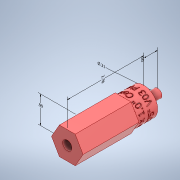
# Autodesk Inventor part: 1x8mmx1_1-inchHexShaft
Saved by Autodesk Inventor 2022.2 (Build 262287010, 287A)
## iProperties
Created: 2020-11-16
Part Number: 1x8mmx1_1-inchHexShaft
Material: PC/ABS Plastic
Document SubType Name: Modeling
Designer: robst
Density: 0.357273 g/cm^3
Appearance: Smooth - Red
Author: robst
Autodesk Inventor part; units mm, degrees
ref_plane "XZ Plane" through (0, 0, 0) normal (0, 1, 0) x (-1, 0, 0)
ref_plane "XY Plane" through (0, 0, 0) normal (0, 0, 1) x (1, 0, 0)
sketch "Sketch1" plane through (0, 0, 0) normal (0, 0, 1) x (1, 0, 0)
  line L0 (14.6647, 0) -> (7.3323, -12.7)
  line L1 (7.3323, -12.7) -> (-7.3323, -12.7)
  line L2 (-7.3323, -12.7) -> (-14.6647, 0)
  line L3 (-14.6647, 0) -> (-7.3323, 12.7)
  line L4 (-7.3323, 12.7) -> (7.3323, 12.7)
  line L5 (7.3323, 12.7) -> (14.6647, 0)
  point P0 (0, 0)
  point P1 (0, 0)
  dimension "d0" = 25.4
  constraints: 12 end point, 1 coincident, 1 horizontal, 13 other
  measures "d0" distance between parallel lines of L1 L4
extrude "Hex Portion" add sketch "Sketch1" along normal mid plane 51.435
sketch "Sketch2" plane through (0, 0, -25.7175) normal (0, 0, -1) x (-1, 0, 0)
  circle A0 centre (0, 0) radius 12.7
  dimension "d3" = 25.4
  constraints: 1 centre point, 1 coincident
  measures "d3" diameter of A0
extrude "Extrusion2" add sketch "Sketch2" along normal blind 19.05
thicken "Reduce Size of Hex Shaft" operation add thickness 0.0953 both sides no extend neighbours yes toward (-0.8660254, -0.5, 0) faces at (10.9985, 6.35, 8.5725) (0, 12.7, 8.5725) (10.9985, -6.35, 8.5725) (0, -12.7, 8.5725) (-10.9985, -6.35, 8.5725) (-10.9985, 6.35, 8.5725)
sketch "Sketch3" plane through (0, 0, -44.7675) normal (0, 0, -1) x (-1, 0, 0)
  circle A0 centre (0, 0) radius 4
  dimension "d14" = 8
  constraints: 1 centre point, 1 coincident
  measures "d14" diameter of A0
extrude "Extrusion3" add sketch "Sketch3" along normal blind 12.7
ref_plane "Work Plane1" through (12.7, 0, -25.7175) normal (1, 0, 0) x (0, 1, 0)
sketch "Sketch4" plane through (12.7, 0, -25.7175) normal (1, 0, 0) x (0, 1, 0)
  line L0 (-12.7, 0) -> (12.7, 0) projected
  line L1 (-12.7, -19.05) -> (12.7, -19.05) projected
  line L2 (-12.7, 0) -> (-12.7, -19.05) construction
  line L3 (-12.7, -9.525) -> (12.7, -9.525) construction
  line L4 (12.7, 0) -> (12.7, -19.05) construction
  line L5 (-33.1661, -6.985) -> (-35.6444, -6.985)
  line L6 (-35.6444, -6.985) -> (-35.6444, -6.4663)
  line L7 (-35.6444, -6.4663) -> (-34.7223, -6.4663)
  line L8 (-34.7223, -6.4663) -> (-34.7223, -3.0618)
  line L9 (-34.7223, -3.0618) -> (-35.6444, -3.0618)
  line L10 (-35.6444, -3.0618) -> (-35.6444, -2.5966)
  spline S0 degree 2 poles (-35.6444, -2.5966) (-35.1216, -2.5966) (-34.6276, -2.3002) (-34.5946, -1.8885) knots 0 0 0 1 2 2 2
  line L11 (-34.5946, -1.8885) -> (-34.0677, -1.8885)
  line L12 (-34.0677, -1.8885) -> (-34.0677, -6.4663)
  line L13 (-34.0677, -6.4663) -> (-33.1661, -6.4663)
  line L14 (-33.1661, -6.4663) -> (-33.1661, -6.985)
  line L15 (-31.4701, -1.6786) -> (-31.6183, -3.6546)
  line L16 (-31.6183, -3.6546) -> (-32.067, -3.6546)
  line L17 (-32.067, -3.6546) -> (-32.2152, -1.6786)
  line L18 (-32.2152, -1.6786) -> (-31.4701, -1.6786)
  line L19 (-30.1857, -1.6786) -> (-30.3339, -3.6546)
  line L20 (-30.3339, -3.6546) -> (-30.7826, -3.6546)
  line L21 (-30.7826, -3.6546) -> (-30.9308, -1.6786)
  line L22 (-30.9308, -1.6786) -> (-30.1857, -1.6786)
  line L23 (-24.1918, -6.985) -> (-24.978, -6.985)
  line L24 (-24.978, -6.985) -> (-25.9043, -5.5524)
  line L25 (-25.9043, -5.5524) -> (-26.8553, -6.985)
  line L26 (-26.8553, -6.985) -> (-27.5839, -6.985)
  line L27 (-27.5839, -6.985) -> (-26.2624, -5.0954)
  line L28 (-26.2624, -5.0954) -> (-27.5716, -3.1729)
  line L29 (-27.5716, -3.1729) -> (-26.7853, -3.1729)
  line L30 (-26.7853, -3.1729) -> (-25.8631, -4.5932)
  line L31 (-25.8631, -4.5932) -> (-24.9204, -3.1729)
  line L32 (-24.9204, -3.1729) -> (-24.1918, -3.1729)
  line L33 (-24.1918, -3.1729) -> (-25.505, -5.0543)
  line L34 (-25.505, -5.0543) -> (-24.1918, -6.985)
  spline S1 degree 2 poles (-20.0709, -7.1003) (-20.4497, -7.1003) (-21.0713, -6.8738) (-21.2895, -6.6639) knots 0 0 0 1 2 2 2
  spline S2 degree 2 poles (-21.2895, -6.6639) (-21.5036, -6.4581) (-21.7259, -5.8982) (-21.7259, -5.5812) knots 0 0 0 1 2 2 2
  spline S3 degree 2 poles (-21.7259, -5.5812) (-21.7259, -5.1695) (-21.2854, -4.4779) (-20.8655, -4.2721) knots 0 0 0 1 2 2 2
  line L35 (-20.8655, -4.2721) -> (-20.8655, -4.2515)
  spline S4 degree 2 poles (-20.8655, -4.2515) (-21.2401, -4.0333) (-21.6024, -3.5146) (-21.6024, -3.1277) knots 0 0 0 1 2 2 2
  spline S5 degree 2 poles (-21.6024, -3.1277) (-21.6024, -2.5554) (-20.7378, -1.7897) (-20.0709, -1.7897) knots 0 0 0 1 2 2 2
  spline S6 degree 2 poles (-20.0709, -1.7897) (-19.3793, -1.7897) (-18.5436, -2.5143) (-18.5436, -3.0824) knots 0 0 0 1 2 2 2
  spline S7 degree 2 poles (-18.5436, -3.0824) (-18.5436, -3.4241) (-18.943, -4.091) (-19.3176, -4.2803) knots 0 0 0 1 2 2 2
  line L36 (-19.3176, -4.2803) -> (-19.3176, -4.3009)
  spline S8 degree 2 poles (-19.3176, -4.3009) (-18.873, -4.5068) (-18.416, -5.0996) (-18.416, -5.5689) knots 0 0 0 1 2 2 2
  spline S9 degree 2 poles (-18.416, -5.5689) (-18.416, -6.2193) (-19.3629, -7.1003) (-20.0709, -7.1003) knots 0 0 0 1 2 2 2
  spline S10 degree 2 poles (-19.1159, -5.6347) (-19.1159, -5.3219) (-19.3629, -4.9514) (-19.7128, -4.762) knots 0 0 0 1 2 2 2
  spline S11 degree 2 poles (-19.7128, -4.762) (-19.8281, -4.6961) (-20.215, -4.5438) (-20.4579, -4.445) knots 0 0 0 1 2 2 2
  spline S12 degree 2 poles (-20.4579, -4.445) (-20.7378, -4.6303) (-21.0384, -5.1819) (-21.0384, -5.5318) knots 0 0 0 1 2 2 2
  spline S13 degree 2 poles (-21.0384, -5.5318) (-21.0384, -5.9929) (-20.4826, -6.5939) (-20.0627, -6.5939) knots 0 0 0 1 2 2 2
  spline S14 degree 2 poles (-20.0627, -6.5939) (-19.6346, -6.5939) (-19.1159, -6.0793) (-19.1159, -5.6347) knots 0 0 0 1 2 2 2
  spline S15 degree 2 poles (-19.2106, -3.0906) (-19.2106, -2.7489) (-19.6675, -2.292) (-20.0751, -2.292) knots 0 0 0 1 2 2 2
  spline S16 degree 2 poles (-20.0751, -2.292) (-20.4456, -2.292) (-20.919, -2.6995) (-20.919, -3.0494) knots 0 0 0 1 2 2 2
  spline S17 degree 2 poles (-20.919, -3.0494) (-20.919, -3.3006) (-20.6761, -3.6505) (-20.4332, -3.7904) knots 0 0 0 1 2 2 2
  spline S18 degree 2 poles (-20.4332, -3.7904) (-20.3303, -3.8481) (-19.8939, -4.0498) (-19.7169, -4.1074) knots 0 0 0 1 2 2 2
  spline S19 degree 2 poles (-19.7169, -4.1074) (-19.4205, -3.881) (-19.2106, -3.3994) (-19.2106, -3.0906) knots 0 0 0 1 2 2 2
  line L37 (-13.3772, -6.985) -> (-13.3772, -4.7785)
  spline S20 degree 2 poles (-13.3772, -4.7785) (-13.3772, -4.515) (-13.4184, -4.0663) (-13.4842, -3.9428) knots 0 0 0 1 2 2 2
  spline S21 degree 2 poles (-13.4842, -3.9428) (-13.5501, -3.8069) (-13.8012, -3.6752) (-14.0194, -3.6752) knots 0 0 0 1 2 2 2
  spline S22 degree 2 poles (-14.0194, -3.6752) (-14.217, -3.6752) (-14.6698, -3.9181) (-14.9086, -4.1486) knots 0 0 0 1 2 2 2
  spline S23 degree 2 poles (-14.9086, -4.1486) (-14.9045, -4.2062) (-14.8963, -4.3668) (-14.8963, -4.4738) knots 0 0 0 1 2 2 2
  line L38 (-14.8963, -4.4738) -> (-14.8963, -6.985)
  line L39 (-14.8963, -6.985) -> (-15.5385, -6.985)
  line L40 (-15.5385, -6.985) -> (-15.5385, -4.7785)
  spline S24 degree 2 poles (-15.5385, -4.7785) (-15.5385, -4.515) (-15.5796, -4.0663) (-15.6455, -3.9428) knots 0 0 0 1 2 2 2
  spline S25 degree 2 poles (-15.6455, -3.9428) (-15.7114, -3.8069) (-15.9625, -3.6752) (-16.1807, -3.6752) knots 0 0 0 1 2 2 2
  spline S26 degree 2 poles (-16.1807, -3.6752) (-16.3865, -3.6752) (-16.8435, -3.9345) (-17.0575, -4.1362) knots 0 0 0 1 2 2 2
  line L41 (-17.0575, -4.1362) -> (-17.0575, -6.985)
  line L42 (-17.0575, -6.985) -> (-17.6997, -6.985)
  line L43 (-17.6997, -6.985) -> (-17.6997, -3.1729)
  line L44 (-17.6997, -3.1729) -> (-17.0575, -3.1729)
  line L45 (-17.0575, -3.1729) -> (-17.0575, -3.5928)
  spline S27 degree 2 poles (-17.0575, -3.5928) (-16.8064, -3.3417) (-16.3124, -3.0659) (-16.016, -3.0659) knots 0 0 0 1 2 2 2
  spline S28 degree 2 poles (-16.016, -3.0659) (-15.6784, -3.0659) (-15.1556, -3.3747) (-15.0198, -3.7246) knots 0 0 0 1 2 2 2
  spline S29 degree 2 poles (-15.0198, -3.7246) (-14.7275, -3.3994) (-14.1758, -3.0659) (-13.8547, -3.0659) knots 0 0 0 1 2 2 2
  spline S30 degree 2 poles (-13.8547, -3.0659) (-13.6077, -3.0659) (-13.2043, -3.2182) (-13.0561, -3.3911) knots 0 0 0 1 2 2 2
  spline S31 degree 2 poles (-13.0561, -3.3911) (-12.9038, -3.564) (-12.735, -4.0827) (-12.735, -4.4738) knots 0 0 0 1 2 2 2
  line L46 (-12.735, -4.4738) -> (-12.735, -6.985)
  line L47 (-12.735, -6.985) -> (-13.3772, -6.985)
  line L48 (-7.5109, -6.985) -> (-7.5109, -4.7785)
  spline S32 degree 2 poles (-7.5109, -4.7785) (-7.5109, -4.515) (-7.5521, -4.0663) (-7.6179, -3.9428) knots 0 0 0 1 2 2 2
  spline S33 degree 2 poles (-7.6179, -3.9428) (-7.6838, -3.8069) (-7.9349, -3.6752) (-8.1531, -3.6752) knots 0 0 0 1 2 2 2
  spline S34 degree 2 poles (-8.1531, -3.6752) (-8.3507, -3.6752) (-8.8036, -3.9181) (-9.0423, -4.1486) knots 0 0 0 1 2 2 2
  spline S35 degree 2 poles (-9.0423, -4.1486) (-9.0382, -4.2062) (-9.03, -4.3668) (-9.03, -4.4738) knots 0 0 0 1 2 2 2
  line L49 (-9.03, -4.4738) -> (-9.03, -6.985)
  line L50 (-9.03, -6.985) -> (-9.6722, -6.985)
  line L51 (-9.6722, -6.985) -> (-9.6722, -4.7785)
  spline S36 degree 2 poles (-9.6722, -4.7785) (-9.6722, -4.515) (-9.7133, -4.0663) (-9.7792, -3.9428) knots 0 0 0 1 2 2 2
  spline S37 degree 2 poles (-9.7792, -3.9428) (-9.8451, -3.8069) (-10.0962, -3.6752) (-10.3144, -3.6752) knots 0 0 0 1 2 2 2
  spline S38 degree 2 poles (-10.3144, -3.6752) (-10.5202, -3.6752) (-10.9772, -3.9345) (-11.1912, -4.1362) knots 0 0 0 1 2 2 2
  line L52 (-11.1912, -4.1362) -> (-11.1912, -6.985)
  line L53 (-11.1912, -6.985) -> (-11.8334, -6.985)
  line L54 (-11.8334, -6.985) -> (-11.8334, -3.1729)
  line L55 (-11.8334, -3.1729) -> (-11.1912, -3.1729)
  line L56 (-11.1912, -3.1729) -> (-11.1912, -3.5928)
  spline S39 degree 2 poles (-11.1912, -3.5928) (-10.9401, -3.3417) (-10.4461, -3.0659) (-10.1497, -3.0659) knots 0 0 0 1 2 2 2
  spline S40 degree 2 poles (-10.1497, -3.0659) (-9.8121, -3.0659) (-9.2893, -3.3747) (-9.1535, -3.7246) knots 0 0 0 1 2 2 2
  spline S41 degree 2 poles (-9.1535, -3.7246) (-8.8612, -3.3994) (-8.3095, -3.0659) (-7.9884, -3.0659) knots 0 0 0 1 2 2 2
  spline S42 degree 2 poles (-7.9884, -3.0659) (-7.7414, -3.0659) (-7.338, -3.2182) (-7.1898, -3.3911) knots 0 0 0 1 2 2 2
  spline S43 degree 2 poles (-7.1898, -3.3911) (-7.0375, -3.564) (-6.8687, -4.0827) (-6.8687, -4.4738) knots 0 0 0 1 2 2 2
  line L57 (-6.8687, -4.4738) -> (-6.8687, -6.985)
  line L58 (-6.8687, -6.985) -> (-7.5109, -6.985)
  line L59 (-0.8254, -6.985) -> (-1.6117, -6.985)
  line L60 (-1.6117, -6.985) -> (-2.5379, -5.5524)
  line L61 (-2.5379, -5.5524) -> (-3.4889, -6.985)
  line L62 (-3.4889, -6.985) -> (-4.2176, -6.985)
  line L63 (-4.2176, -6.985) -> (-2.8961, -5.0954)
  line L64 (-2.8961, -5.0954) -> (-4.2052, -3.1729)
  line L65 (-4.2052, -3.1729) -> (-3.4189, -3.1729)
  line L66 (-3.4189, -3.1729) -> (-2.4968, -4.5932)
  line L67 (-2.4968, -4.5932) -> (-1.5541, -3.1729)
  line L68 (-1.5541, -3.1729) -> (-0.8254, -3.1729)
  line L69 (-0.8254, -3.1729) -> (-2.1386, -5.0543)
  line L70 (-2.1386, -5.0543) -> (-0.8254, -6.985)
  line L71 (4.6375, -6.985) -> (2.1592, -6.985)
  line L72 (2.1592, -6.985) -> (2.1592, -6.4663)
  line L73 (2.1592, -6.4663) -> (3.0813, -6.4663)
  line L74 (3.0813, -6.4663) -> (3.0813, -3.0618)
  line L75 (3.0813, -3.0618) -> (2.1592, -3.0618)
  line L76 (2.1592, -3.0618) -> (2.1592, -2.5966)
  spline S44 degree 2 poles (2.1592, -2.5966) (2.682, -2.5966) (3.176, -2.3002) (3.209, -1.8885) knots 0 0 0 1 2 2 2
  line L77 (3.209, -1.8885) -> (3.7359, -1.8885)
  line L78 (3.7359, -1.8885) -> (3.7359, -6.4663)
  line L79 (3.7359, -6.4663) -> (4.6375, -6.4663)
  line L80 (4.6375, -6.4663) -> (4.6375, -6.985)
  line L81 (6.6629, -6.985) -> (5.8478, -6.985)
  line L82 (5.8478, -6.985) -> (5.8478, -6.0135)
  line L83 (5.8478, -6.0135) -> (6.6629, -6.0135)
  line L84 (6.6629, -6.0135) -> (6.6629, -6.985)
  spline S45 degree 2 poles (10.8495, -4.445) (10.8495, -5.8117) (10.055, -7.092) (9.2276, -7.092) knots 0 0 0 1 2 2 2
  spline S46 degree 2 poles (9.2276, -7.092) (8.3878, -7.092) (7.6015, -5.787) (7.6015, -4.4491) knots 0 0 0 1 2 2 2
  spline S47 degree 2 poles (7.6015, -4.4491) (7.6015, -3.0741) (8.396, -1.8021) (9.2276, -1.8021) knots 0 0 0 1 2 2 2
  spline S48 degree 2 poles (9.2276, -1.8021) (10.0633, -1.8021) (10.8495, -3.1194) (10.8495, -4.445) knots 0 0 0 1 2 2 2
  spline S49 degree 2 poles (9.9768, -5.9929) (10.0756, -5.7418) (10.1579, -4.9678) (10.1579, -4.445) knots 0 0 0 1 2 2 2
  spline S50 degree 2 poles (10.1579, -4.445) (10.1579, -3.9222) (10.0756, -3.1524) (9.9727, -2.893) knots 0 0 0 1 2 2 2
  spline S51 degree 2 poles (9.9727, -2.893) (9.8698, -2.6337) (9.5116, -2.3661) (9.2276, -2.3661) knots 0 0 0 1 2 2 2
  spline S52 degree 2 poles (9.2276, -2.3661) (8.9435, -2.3661) (8.5771, -2.6337) (8.4701, -2.9012) knots 0 0 0 1 2 2 2
  spline S53 degree 2 poles (8.4701, -2.9012) (8.3672, -3.1606) (8.2931, -3.951) (8.2931, -4.4491) knots 0 0 0 1 2 2 2
  spline S54 degree 2 poles (8.2931, -4.4491) (8.2931, -4.9843) (8.3589, -5.7006) (8.466, -5.9805) knots 0 0 0 1 2 2 2
  spline S55 degree 2 poles (8.466, -5.9805) (8.5648, -6.244) (8.9312, -6.528) (9.2276, -6.528) knots 0 0 0 1 2 2 2
  spline S56 degree 2 poles (9.2276, -6.528) (9.5075, -6.528) (9.8739, -6.2605) (9.9768, -5.9929) knots 0 0 0 1 2 2 2
  line L85 (12.2616, -1.6786) -> (12.1134, -3.6546)
  line L86 (12.1134, -3.6546) -> (11.6647, -3.6546)
  line L87 (11.6647, -3.6546) -> (11.5164, -1.6786)
  line L88 (11.5164, -1.6786) -> (12.2616, -1.6786)
  line L89 (13.546, -1.6786) -> (13.3978, -3.6546)
  line L90 (13.3978, -3.6546) -> (12.9491, -3.6546)
  line L91 (12.9491, -3.6546) -> (12.8009, -1.6786)
  line L92 (12.8009, -1.6786) -> (13.546, -1.6786)
  spline S57 degree 2 poles (18.6136, -7.0756) (18.1196, -7.0756) (17.2839, -6.7421) (16.9793, -6.4087) knots 0 0 0 1 2 2 2
  spline S58 degree 2 poles (16.9793, -6.4087) (16.6747, -6.0793) (16.3412, -5.0913) (16.3412, -4.4491) knots 0 0 0 1 2 2 2
  spline S59 degree 2 poles (16.3412, -4.4491) (16.3412, -3.811) (16.6664, -2.8642) (16.9752, -2.5143) knots 0 0 0 1 2 2 2
  spline S60 degree 2 poles (16.9752, -2.5143) (17.2798, -2.1726) (18.1114, -1.8144) (18.626, -1.8144) knots 0 0 0 1 2 2 2
  spline S61 degree 2 poles (18.626, -1.8144) (18.8812, -1.8144) (19.3299, -1.8885) (19.5193, -1.9462) knots 0 0 0 1 2 2 2
  spline S62 degree 2 poles (19.5193, -1.9462) (19.684, -1.9997) (20.0257, -2.152) (20.1944, -2.2426) knots 0 0 0 1 2 2 2
  line L93 (20.1944, -2.2426) -> (20.1944, -3.0577)
  line L94 (20.1944, -3.0577) -> (20.1409, -3.0577)
  spline S63 degree 2 poles (20.1409, -3.0577) (20.0504, -2.9753) (19.7704, -2.7448) (19.5687, -2.6337) knots 0 0 0 1 2 2 2
  spline S64 degree 2 poles (19.5687, -2.6337) (19.3752, -2.5266) (18.9183, -2.3908) (18.6219, -2.3908) knots 0 0 0 1 2 2 2
  spline S65 degree 2 poles (18.6219, -2.3908) (18.2966, -2.3908) (17.7162, -2.6584) (17.498, -2.9136) knots 0 0 0 1 2 2 2
  spline S66 degree 2 poles (17.498, -2.9136) (17.2839, -3.1729) (17.0452, -3.9592) (17.0452, -4.4491) knots 0 0 0 1 2 2 2
  spline S67 degree 2 poles (17.0452, -4.4491) (17.0452, -4.9719) (17.2963, -5.7253) (17.5145, -5.9846) knots 0 0 0 1 2 2 2
  spline S68 degree 2 poles (17.5145, -5.9846) (17.7285, -6.2358) (18.3008, -6.491) (18.6219, -6.491) knots 0 0 0 1 2 2 2
  spline S69 degree 2 poles (18.6219, -6.491) (18.9141, -6.491) (19.4123, -6.3469) (19.6058, -6.2399) knots 0 0 0 1 2 2 2
  spline S70 degree 2 poles (19.6058, -6.2399) (19.791, -6.1328) (20.0668, -5.9105) (20.145, -5.8323) knots 0 0 0 1 2 2 2
  line L95 (20.145, -5.8323) -> (20.1944, -5.8323)
  line L96 (20.1944, -5.8323) -> (20.1944, -6.6392)
  spline S71 degree 2 poles (20.1944, -6.6392) (20.0257, -6.7174) (19.7293, -6.8615) (19.5193, -6.9274) knots 0 0 0 1 2 2 2
  spline S72 degree 2 poles (19.5193, -6.9274) (19.297, -7.0015) (18.9183, -7.0756) (18.6136, -7.0756) knots 0 0 0 1 2 2 2
  spline S73 degree 2 poles (22.4298, -7.0715) (21.5159, -7.0715) (20.5114, -6.0464) (20.5114, -5.0996) knots 0 0 0 1 2 2 2
  spline S74 degree 2 poles (20.5114, -5.0996) (20.5114, -4.1692) (21.4871, -3.0659) (22.2734, -3.0659) knots 0 0 0 1 2 2 2
  spline S75 degree 2 poles (22.2734, -3.0659) (22.6274, -3.0659) (23.1749, -3.2717) (23.3766, -3.4899) knots 0 0 0 1 2 2 2
  spline S76 degree 2 poles (23.3766, -3.4899) (23.5825, -3.7081) (23.8007, -4.338) (23.8007, -4.7949) knots 0 0 0 1 2 2 2
  line L97 (23.8007, -4.7949) -> (23.8007, -5.1448)
  line L98 (23.8007, -5.1448) -> (21.1619, -5.1448)
  spline S77 degree 2 poles (21.1619, -5.1448) (21.1619, -5.8076) (21.8288, -6.5116) (22.4216, -6.5116) knots 0 0 0 1 2 2 2
  spline S78 degree 2 poles (22.4216, -6.5116) (22.6315, -6.5116) (23.0391, -6.4169) (23.2037, -6.3428) knots 0 0 0 1 2 2 2
  spline S79 degree 2 poles (23.2037, -6.3428) (23.3766, -6.2605) (23.6154, -6.1164) (23.6936, -6.0505) knots 0 0 0 1 2 2 2
  line L99 (23.6936, -6.0505) -> (23.7307, -6.0505)
  line L100 (23.7307, -6.0505) -> (23.7307, -6.7503)
  spline S80 degree 2 poles (23.7307, -6.7503) (23.6195, -6.7956) (23.282, -6.9274) (23.1502, -6.9644) knots 0 0 0 1 2 2 2
  spline S81 degree 2 poles (23.1502, -6.9644) (22.965, -7.0179) (22.6603, -7.0715) (22.4298, -7.0715) knots 0 0 0 1 2 2 2
  spline S82 degree 2 poles (23.1749, -4.655) (23.1667, -4.3956) (23.0597, -4.0169) (22.9567, -3.8892) knots 0 0 0 1 2 2 2
  spline S83 degree 2 poles (22.9567, -3.8892) (22.8456, -3.7452) (22.4957, -3.5928) (22.2363, -3.5928) knots 0 0 0 1 2 2 2
  spline S84 degree 2 poles (22.2363, -3.5928) (21.9811, -3.5928) (21.6229, -3.7452) (21.4747, -3.8934) knots 0 0 0 1 2 2 2
  spline S85 degree 2 poles (21.4747, -3.8934) (21.3306, -4.0457) (21.1824, -4.4121) (21.1619, -4.655) knots 0 0 0 1 2 2 2
  line L101 (21.1619, -4.655) -> (23.1749, -4.655)
  line L102 (27.4439, -6.985) -> (26.8017, -6.985)
  line L103 (26.8017, -6.985) -> (26.8017, -4.8114)
  spline S86 degree 2 poles (26.8017, -4.8114) (26.8017, -4.5479) (26.7523, -4.0951) (26.6782, -3.9592) knots 0 0 0 1 2 2 2
  spline S87 degree 2 poles (26.6782, -3.9592) (26.6, -3.8151) (26.3201, -3.6752) (26.0813, -3.6752) knots 0 0 0 1 2 2 2
  spline S88 degree 2 poles (26.0813, -3.6752) (25.8425, -3.6752) (25.3362, -3.9304) (25.0933, -4.1362) knots 0 0 0 1 2 2 2
  line L104 (25.0933, -4.1362) -> (25.0933, -6.985)
  line L105 (25.0933, -6.985) -> (24.4511, -6.985)
  line L106 (24.4511, -6.985) -> (24.4511, -3.1729)
  line L107 (24.4511, -3.1729) -> (25.0933, -3.1729)
  line L108 (25.0933, -3.1729) -> (25.0933, -3.597)
  spline S89 degree 2 poles (25.0933, -3.597) (25.3815, -3.3376) (25.9372, -3.0659) (26.2501, -3.0659) knots 0 0 0 1 2 2 2
  spline S90 degree 2 poles (26.2501, -3.0659) (26.81, -3.0659) (27.4439, -3.8069) (27.4439, -4.5109) knots 0 0 0 1 2 2 2
  line L109 (27.4439, -4.5109) -> (27.4439, -6.985)
  spline S91 degree 2 poles (29.4982, -7.0591) (28.9753, -7.0591) (28.3867, -6.4622) (28.3867, -5.8159) knots 0 0 0 1 2 2 2
  line L110 (28.3867, -5.8159) -> (28.3867, -3.704)
  line L111 (28.3867, -3.704) -> (27.9544, -3.704)
  line L112 (27.9544, -3.704) -> (27.9544, -3.1729)
  line L113 (27.9544, -3.1729) -> (28.3867, -3.1729)
  line L114 (28.3867, -3.1729) -> (28.3867, -2.0779)
  line L115 (28.3867, -2.0779) -> (29.0289, -2.0779)
  line L116 (29.0289, -2.0779) -> (29.0289, -3.1729)
  line L117 (29.0289, -3.1729) -> (30.2104, -3.1729)
  line L118 (30.2104, -3.1729) -> (30.2104, -3.704)
  line L119 (30.2104, -3.704) -> (29.0289, -3.704)
  line L120 (29.0289, -3.704) -> (29.0289, -5.5195)
  spline S92 degree 2 poles (29.0289, -5.5195) (29.0289, -5.8076) (29.0494, -6.1246) (29.1194, -6.2605) knots 0 0 0 1 2 2 2
  spline S93 degree 2 poles (29.1194, -6.2605) (29.1771, -6.3798) (29.4364, -6.4992) (29.6587, -6.4992) knots 0 0 0 1 2 2 2
  spline S94 degree 2 poles (29.6587, -6.4992) (29.8152, -6.4992) (30.1074, -6.4045) (30.1733, -6.3757) knots 0 0 0 1 2 2 2
  line L121 (30.1733, -6.3757) -> (30.2104, -6.3757)
  line L122 (30.2104, -6.3757) -> (30.2104, -6.9521)
  spline S95 degree 2 poles (30.2104, -6.9521) (30.0292, -7.0015) (29.6587, -7.0591) (29.4982, -7.0591) knots 0 0 0 1 2 2 2
  spline S96 degree 2 poles (32.3387, -7.0715) (31.4248, -7.0715) (30.4203, -6.0464) (30.4203, -5.0996) knots 0 0 0 1 2 2 2
  spline S97 degree 2 poles (30.4203, -5.0996) (30.4203, -4.1692) (31.396, -3.0659) (32.1823, -3.0659) knots 0 0 0 1 2 2 2
  spline S98 degree 2 poles (32.1823, -3.0659) (32.5363, -3.0659) (33.0838, -3.2717) (33.2855, -3.4899) knots 0 0 0 1 2 2 2
  spline S99 degree 2 poles (33.2855, -3.4899) (33.4914, -3.7081) (33.7095, -4.338) (33.7095, -4.7949) knots 0 0 0 1 2 2 2
  line L123 (33.7095, -4.7949) -> (33.7095, -5.1448)
  line L124 (33.7095, -5.1448) -> (31.0707, -5.1448)
  spline S100 degree 2 poles (31.0707, -5.1448) (31.0707, -5.8076) (31.7376, -6.5116) (32.3305, -6.5116) knots 0 0 0 1 2 2 2
  spline S101 degree 2 poles (32.3305, -6.5116) (32.5404, -6.5116) (32.948, -6.4169) (33.1126, -6.3428) knots 0 0 0 1 2 2 2
  spline S102 degree 2 poles (33.1126, -6.3428) (33.2855, -6.2605) (33.5243, -6.1164) (33.6025, -6.0505) knots 0 0 0 1 2 2 2
  line L125 (33.6025, -6.0505) -> (33.6396, -6.0505)
  line L126 (33.6396, -6.0505) -> (33.6396, -6.7503)
  spline S103 degree 2 poles (33.6396, -6.7503) (33.5284, -6.7956) (33.1908, -6.9274) (33.0591, -6.9644) knots 0 0 0 1 2 2 2
  spline S104 degree 2 poles (33.0591, -6.9644) (32.8739, -7.0179) (32.5692, -7.0715) (32.3387, -7.0715) knots 0 0 0 1 2 2 2
  spline S105 degree 2 poles (33.0838, -4.655) (33.0756, -4.3956) (32.9685, -4.0169) (32.8656, -3.8892) knots 0 0 0 1 2 2 2
  spline S106 degree 2 poles (32.8656, -3.8892) (32.7545, -3.7452) (32.4046, -3.5928) (32.1452, -3.5928) knots 0 0 0 1 2 2 2
  spline S107 degree 2 poles (32.1452, -3.5928) (31.89, -3.5928) (31.5318, -3.7452) (31.3836, -3.8934) knots 0 0 0 1 2 2 2
  spline S108 degree 2 poles (31.3836, -3.8934) (31.2395, -4.0457) (31.0913, -4.4121) (31.0707, -4.655) knots 0 0 0 1 2 2 2
  line L127 (31.0707, -4.655) -> (33.0838, -4.655)
  line L128 (36.3813, -3.8604) -> (36.3483, -3.8604)
  spline S109 degree 2 poles (36.3483, -3.8604) (36.2742, -3.8398) (36.1137, -3.8316) (36.0025, -3.8316) knots 0 0 0 1 2 2 2
  spline S110 degree 2 poles (36.0025, -3.8316) (35.7432, -3.8316) (35.2327, -4.058) (35.0022, -4.2803) knots 0 0 0 1 2 2 2
  line L129 (35.0022, -4.2803) -> (35.0022, -6.985)
  line L130 (35.0022, -6.985) -> (34.36, -6.985)
  line L131 (34.36, -6.985) -> (34.36, -3.1729)
  line L132 (34.36, -3.1729) -> (35.0022, -3.1729)
  line L133 (35.0022, -3.1729) -> (35.0022, -3.741)
  spline S111 degree 2 poles (35.0022, -3.741) (35.3521, -3.4282) (35.8749, -3.1729) (36.1219, -3.1729) knots 0 0 0 1 2 2 2
  spline S112 degree 2 poles (36.1219, -3.1729) (36.2207, -3.1729) (36.3195, -3.1812) (36.3813, -3.1935) knots 0 0 0 1 2 2 2
  line L134 (36.3813, -3.1935) -> (36.3813, -3.8604)
  spline S113 degree 2 poles (-33.1538, -15.6168) (-33.7054, -15.6168) (-34.4794, -15.3863) (-34.8211, -15.2216) knots 0 0 0 1 2 2 2
  line L135 (-34.8211, -15.2216) -> (-34.8211, -14.3735)
  line L136 (-34.8211, -14.3735) -> (-34.7717, -14.3735)
  spline S114 degree 2 poles (-34.7717, -14.3735) (-34.4382, -14.6864) (-33.5943, -15.0322) (-33.2032, -15.0322) knots 0 0 0 1 2 2 2
  spline S115 degree 2 poles (-33.2032, -15.0322) (-32.6433, -15.0322) (-32.0711, -14.567) (-32.0711, -14.1842) knots 0 0 0 1 2 2 2
  spline S116 degree 2 poles (-32.0711, -14.1842) (-32.0711, -13.8795) (-32.3716, -13.5008) (-32.6968, -13.4061) knots 0 0 0 1 2 2 2
  spline S117 degree 2 poles (-32.6968, -13.4061) (-32.9315, -13.3403) (-33.3226, -13.2497) (-33.6149, -13.1756) knots 0 0 0 1 2 2 2
  spline S118 degree 2 poles (-33.6149, -13.1756) (-33.8783, -13.1056) (-34.2941, -12.8957) (-34.4547, -12.7269) knots 0 0 0 1 2 2 2
  spline S119 degree 2 poles (-34.4547, -12.7269) (-34.6111, -12.5581) (-34.784, -12.1053) (-34.784, -11.8088) knots 0 0 0 1 2 2 2
  spline S120 degree 2 poles (-34.784, -11.8088) (-34.784, -11.1913) (-33.8207, -10.3557) (-33.0756, -10.3557) knots 0 0 0 1 2 2 2
  spline S121 degree 2 poles (-33.0756, -10.3557) (-32.6474, -10.3557) (-31.89, -10.5244) (-31.5647, -10.685) knots 0 0 0 1 2 2 2
  line L137 (-31.5647, -10.685) -> (-31.5647, -11.4919)
  line L138 (-31.5647, -11.4919) -> (-31.6141, -11.4919)
  spline S122 degree 2 poles (-31.6141, -11.4919) (-31.857, -11.2696) (-32.6145, -10.9402) (-33.0303, -10.9402) knots 0 0 0 1 2 2 2
  spline S123 degree 2 poles (-33.0303, -10.9402) (-33.4996, -10.9402) (-34.08, -11.3807) (-34.08, -11.7389) knots 0 0 0 1 2 2 2
  spline S124 degree 2 poles (-34.08, -11.7389) (-34.08, -12.06) (-33.7384, -12.4428) (-33.4173, -12.5293) knots 0 0 0 1 2 2 2
  spline S125 degree 2 poles (-33.4173, -12.5293) (-33.2032, -12.5869) (-32.5816, -12.7351) (-32.3757, -12.7969) knots 0 0 0 1 2 2 2
  spline S126 degree 2 poles (-32.3757, -12.7969) (-31.8529, -12.9574) (-31.3671, -13.6037) (-31.3671, -14.0771) knots 0 0 0 1 2 2 2
  spline S127 degree 2 poles (-31.3671, -14.0771) (-31.3671, -14.3777) (-31.61, -14.954) (-31.8282, -15.1557) knots 0 0 0 1 2 2 2
  spline S128 degree 2 poles (-31.8282, -15.1557) (-32.0711, -15.378) (-32.6886, -15.6168) (-33.1538, -15.6168) knots 0 0 0 1 2 2 2
  line L139 (-27.7362, -15.5262) -> (-28.3784, -15.5262)
  line L140 (-28.3784, -15.5262) -> (-28.3784, -13.3526)
  spline S129 degree 2 poles (-28.3784, -13.3526) (-28.3784, -13.0891) (-28.4278, -12.6363) (-28.5019, -12.5005) knots 0 0 0 1 2 2 2
  spline S130 degree 2 poles (-28.5019, -12.5005) (-28.5801, -12.3564) (-28.8601, -12.2164) (-29.0988, -12.2164) knots 0 0 0 1 2 2 2
  spline S131 degree 2 poles (-29.0988, -12.2164) (-29.3376, -12.2164) (-29.844, -12.4716) (-30.0869, -12.6775) knots 0 0 0 1 2 2 2
  line L141 (-30.0869, -12.6775) -> (-30.0869, -15.5262)
  line L142 (-30.0869, -15.5262) -> (-30.7291, -15.5262)
  line L143 (-30.7291, -15.5262) -> (-30.7291, -10.2198)
  line L144 (-30.7291, -10.2198) -> (-30.0869, -10.2198)
  line L145 (-30.0869, -10.2198) -> (-30.0869, -12.1382)
  spline S132 degree 2 poles (-30.0869, -12.1382) (-29.7987, -11.8788) (-29.2429, -11.6071) (-28.9301, -11.6071) knots 0 0 0 1 2 2 2
  spline S133 degree 2 poles (-28.9301, -11.6071) (-28.3702, -11.6071) (-27.7362, -12.3481) (-27.7362, -13.0521) knots 0 0 0 1 2 2 2
  line L146 (-27.7362, -13.0521) -> (-27.7362, -15.5262)
  spline S134 degree 2 poles (-24.7105, -15.1228) (-24.7887, -15.1804) (-25.0521, -15.3863) (-25.1756, -15.448) knots 0 0 0 1 2 2 2
  spline S135 degree 2 poles (-25.1756, -15.448) (-25.3444, -15.5386) (-25.6614, -15.6333) (-25.9496, -15.6333) knots 0 0 0 1 2 2 2
  spline S136 degree 2 poles (-25.9496, -15.6333) (-26.1842, -15.6333) (-26.6082, -15.4562) (-26.7688, -15.2957) knots 0 0 0 1 2 2 2
  spline S137 degree 2 poles (-26.7688, -15.2957) (-26.9211, -15.1393) (-27.1064, -14.6782) (-27.1064, -14.4229) knots 0 0 0 1 2 2 2
  spline S138 degree 2 poles (-27.1064, -14.4229) (-27.1064, -14.0277) (-26.7729, -13.4679) (-26.4106, -13.3073) knots 0 0 0 1 2 2 2
  spline S139 degree 2 poles (-26.4106, -13.3073) (-26.0895, -13.1591) (-25.2168, -13.048) (-24.7105, -13.0192) knots 0 0 0 1 2 2 2
  line L147 (-24.7105, -13.0192) -> (-24.7105, -12.8957)
  spline S140 degree 2 poles (-24.7105, -12.8957) (-24.7105, -12.6734) (-24.8463, -12.3975) (-24.9698, -12.3193) knots 0 0 0 1 2 2 2
  spline S141 degree 2 poles (-24.9698, -12.3193) (-25.0933, -12.2411) (-25.4473, -12.1917) (-25.6367, -12.1917) knots 0 0 0 1 2 2 2
  spline S142 degree 2 poles (-25.6367, -12.1917) (-25.859, -12.1917) (-26.46, -12.3234) (-26.7606, -12.4511) knots 0 0 0 1 2 2 2
  line L148 (-26.7606, -12.4511) -> (-26.7976, -12.4511)
  line L149 (-26.7976, -12.4511) -> (-26.7976, -11.7965)
  spline S143 degree 2 poles (-26.7976, -11.7965) (-26.6206, -11.7471) (-25.9578, -11.6236) (-25.6326, -11.6236) knots 0 0 0 1 2 2 2
  spline S144 degree 2 poles (-25.6326, -11.6236) (-25.2374, -11.6236) (-24.6981, -11.7471) (-24.484, -11.9076) knots 0 0 0 1 2 2 2
  spline S145 degree 2 poles (-24.484, -11.9076) (-24.2741, -12.0641) (-24.0682, -12.5622) (-24.0682, -12.9204) knots 0 0 0 1 2 2 2
  line L150 (-24.0682, -12.9204) -> (-24.0682, -15.5262)
  line L151 (-24.0682, -15.5262) -> (-24.7105, -15.5262)
  line L152 (-24.7105, -15.5262) -> (-24.7105, -15.1228)
  line L153 (-24.7105, -14.5876) -> (-24.7105, -13.5296)
  spline S146 degree 2 poles (-24.7105, -13.5296) (-24.941, -13.5502) (-25.6367, -13.6202) (-25.8549, -13.6861) knots 0 0 0 1 2 2 2
  spline S147 degree 2 poles (-25.8549, -13.6861) (-26.1101, -13.7643) (-26.4436, -14.0895) (-26.4436, -14.3777) knots 0 0 0 1 2 2 2
  spline S148 degree 2 poles (-26.4436, -14.3777) (-26.4436, -14.707) (-26.0731, -15.0405) (-25.719, -15.0405) knots 0 0 0 1 2 2 2
  spline S149 degree 2 poles (-25.719, -15.0405) (-25.4185, -15.0405) (-24.9245, -14.7811) (-24.7105, -14.5876) knots 0 0 0 1 2 2 2
  line L154 (-21.1619, -10.8373) -> (-21.1948, -10.8373)
  spline S150 degree 2 poles (-21.1948, -10.8373) (-21.2812, -10.8044) (-21.6023, -10.7467) (-21.73, -10.7467) knots 0 0 0 1 2 2 2
  spline S151 degree 2 poles (-21.73, -10.7467) (-22.1334, -10.7467) (-22.4792, -11.109) (-22.4792, -11.5865) knots 0 0 0 1 2 2 2
  line L155 (-22.4792, -11.5865) -> (-22.4792, -11.7142)
  line L156 (-22.4792, -11.7142) -> (-21.4171, -11.7142)
  line L157 (-21.4171, -11.7142) -> (-21.4171, -12.2452)
  line L158 (-21.4171, -12.2452) -> (-22.4586, -12.2452)
  line L159 (-22.4586, -12.2452) -> (-22.4586, -15.5262)
  line L160 (-22.4586, -15.5262) -> (-23.1008, -15.5262)
  line L161 (-23.1008, -15.5262) -> (-23.1008, -12.2452)
  line L162 (-23.1008, -12.2452) -> (-23.5331, -12.2452)
  line L163 (-23.5331, -12.2452) -> (-23.5331, -11.7142)
  line L164 (-23.5331, -11.7142) -> (-23.1008, -11.7142)
  line L165 (-23.1008, -11.7142) -> (-23.1008, -11.5865)
  spline S152 degree 2 poles (-23.1008, -11.5865) (-23.1008, -10.9032) (-22.438, -10.1869) (-21.8205, -10.1869) knots 0 0 0 1 2 2 2
  spline S153 degree 2 poles (-21.8205, -10.1869) (-21.6435, -10.1869) (-21.3018, -10.2239) (-21.1619, -10.2486) knots 0 0 0 1 2 2 2
  line L166 (-21.1619, -10.2486) -> (-21.1619, -10.8373)
  spline S154 degree 2 poles (-19.6428, -15.6003) (-20.1656, -15.6003) (-20.7543, -15.0034) (-20.7543, -14.3571) knots 0 0 0 1 2 2 2
  line L167 (-20.7543, -14.3571) -> (-20.7543, -12.2452)
  line L168 (-20.7543, -12.2452) -> (-21.1866, -12.2452)
  line L169 (-21.1866, -12.2452) -> (-21.1866, -11.7142)
  line L170 (-21.1866, -11.7142) -> (-20.7543, -11.7142)
  line L171 (-20.7543, -11.7142) -> (-20.7543, -10.6191)
  line L172 (-20.7543, -10.6191) -> (-20.1121, -10.6191)
  line L173 (-20.1121, -10.6191) -> (-20.1121, -11.7142)
  line L174 (-20.1121, -11.7142) -> (-18.9306, -11.7142)
  line L175 (-18.9306, -11.7142) -> (-18.9306, -12.2452)
  line L176 (-18.9306, -12.2452) -> (-20.1121, -12.2452)
  line L177 (-20.1121, -12.2452) -> (-20.1121, -14.0607)
  spline S155 degree 2 poles (-20.1121, -14.0607) (-20.1121, -14.3488) (-20.0915, -14.6658) (-20.0215, -14.8017) knots 0 0 0 1 2 2 2
  spline S156 degree 2 poles (-20.0215, -14.8017) (-19.9639, -14.9211) (-19.7046, -15.0405) (-19.4823, -15.0405) knots 0 0 0 1 2 2 2
  spline S157 degree 2 poles (-19.4823, -15.0405) (-19.3258, -15.0405) (-19.0335, -14.9458) (-18.9677, -14.917) knots 0 0 0 1 2 2 2
  line L178 (-18.9677, -14.917) -> (-18.9306, -14.917)
  line L179 (-18.9306, -14.917) -> (-18.9306, -15.4933)
  spline S158 degree 2 poles (-18.9306, -15.4933) (-19.1117, -15.5427) (-19.4823, -15.6003) (-19.6428, -15.6003) knots 0 0 0 1 2 2 2
  spline S159 degree 2 poles (-14.9992, -10.9279) (-15.1844, -10.9279) (-15.5508, -11.0184) (-15.7278, -11.0884) knots 0 0 0 1 2 2 2
  spline S160 degree 2 poles (-15.7278, -11.0884) (-15.8925, -11.1584) (-16.1354, -11.3066) (-16.2301, -11.3725) knots 0 0 0 1 2 2 2
  line L180 (-16.2301, -11.3725) -> (-16.2712, -11.3725)
  line L181 (-16.2712, -11.3725) -> (-16.2712, -10.6521)
  spline S161 degree 2 poles (-16.2712, -10.6521) (-16.0489, -10.5327) (-15.2873, -10.3392) (-14.9457, -10.3392) knots 0 0 0 1 2 2 2
  spline S162 degree 2 poles (-14.9457, -10.3392) (-14.5999, -10.3392) (-14.0853, -10.4792) (-13.8753, -10.6274) knots 0 0 0 1 2 2 2
  spline S163 degree 2 poles (-13.8753, -10.6274) (-13.653, -10.7879) (-13.4225, -11.2531) (-13.4225, -11.566) knots 0 0 0 1 2 2 2
  spline S164 degree 2 poles (-13.4225, -11.566) (-13.4225, -11.9859) (-13.9741, -12.6198) (-14.3611, -12.7022) knots 0 0 0 1 2 2 2
  line L182 (-14.3611, -12.7022) -> (-14.3611, -12.7516)
  spline S165 degree 2 poles (-14.3611, -12.7516) (-14.2005, -12.7845) (-13.8341, -12.9327) (-13.6777, -13.0809) knots 0 0 0 1 2 2 2
  spline S166 degree 2 poles (-13.6777, -13.0809) (-13.5213, -13.225) (-13.3237, -13.6861) (-13.3237, -14.0195) knots 0 0 0 1 2 2 2
  spline S167 degree 2 poles (-13.3237, -14.0195) (-13.3237, -14.3612) (-13.5583, -14.9417) (-13.7724, -15.164) knots 0 0 0 1 2 2 2
  spline S168 degree 2 poles (-13.7724, -15.164) (-13.9947, -15.3945) (-14.6246, -15.6333) (-15.0239, -15.6333) knots 0 0 0 1 2 2 2
  spline S169 degree 2 poles (-15.0239, -15.6333) (-15.4067, -15.6333) (-16.156, -15.448) (-16.4112, -15.3204) knots 0 0 0 1 2 2 2
  line L183 (-16.4112, -15.3204) -> (-16.4112, -14.6)
  line L184 (-16.4112, -14.6) -> (-16.3618, -14.6)
  spline S170 degree 2 poles (-16.3618, -14.6) (-16.1477, -14.7564) (-15.4232, -15.0446) (-15.065, -15.0446) knots 0 0 0 1 2 2 2
  spline S171 degree 2 poles (-15.065, -15.0446) (-14.8551, -15.0446) (-14.4352, -14.9128) (-14.2952, -14.7605) knots 0 0 0 1 2 2 2
  spline S172 degree 2 poles (-14.2952, -14.7605) (-14.1594, -14.6082) (-14.0153, -14.2459) (-14.0153, -13.9701) knots 0 0 0 1 2 2 2
  spline S173 degree 2 poles (-14.0153, -13.9701) (-14.0153, -13.6943) (-14.1758, -13.3361) (-14.3199, -13.2332) knots 0 0 0 1 2 2 2
  spline S174 degree 2 poles (-14.3199, -13.2332) (-14.464, -13.1303) (-14.8551, -13.0521) (-15.0856, -13.0521) knots 0 0 0 1 2 2 2
  line L185 (-15.0856, -13.0521) -> (-15.3738, -13.0521)
  line L186 (-15.3738, -13.0521) -> (-15.3738, -12.4881)
  line L187 (-15.3738, -12.4881) -> (-15.1474, -12.4881)
  spline S175 degree 2 poles (-15.1474, -12.4881) (-14.6904, -12.4881) (-14.1141, -12.0517) (-14.1141, -11.6359) knots 0 0 0 1 2 2 2
  spline S176 degree 2 poles (-14.1141, -11.6359) (-14.1141, -11.4425) (-14.2623, -11.1666) (-14.3817, -11.0843) knots 0 0 0 1 2 2 2
  spline S177 degree 2 poles (-14.3817, -11.0843) (-14.5093, -10.9979) (-14.8222, -10.9279) (-14.9992, -10.9279) knots 0 0 0 1 2 2 2
  line L188 (-11.467, -15.5262) -> (-12.2822, -15.5262)
  line L189 (-12.2822, -15.5262) -> (-12.2822, -14.5547)
  line L190 (-12.2822, -14.5547) -> (-11.467, -14.5547)
  line L191 (-11.467, -14.5547) -> (-11.467, -15.5262)
  line L192 (-7.3092, -15.5262) -> (-10.442, -15.5262)
  line L193 (-10.442, -15.5262) -> (-10.442, -14.8058)
  spline S178 degree 2 poles (-10.442, -14.8058) (-10.1044, -14.4888) (-9.5034, -13.9001) (-9.2152, -13.5831) knots 0 0 0 1 2 2 2
  spline S179 degree 2 poles (-9.2152, -13.5831) (-8.6348, -12.9451) (-8.2107, -12.1794) (-8.2107, -11.7718) knots 0 0 0 1 2 2 2
  spline S180 degree 2 poles (-8.2107, -11.7718) (-8.2107, -11.5577) (-8.3425, -11.2366) (-8.4619, -11.1337) knots 0 0 0 1 2 2 2
  spline S181 degree 2 poles (-8.4619, -11.1337) (-8.5812, -11.0308) (-8.8941, -10.9279) (-9.0835, -10.9279) knots 0 0 0 1 2 2 2
  spline S182 degree 2 poles (-9.0835, -10.9279) (-9.2646, -10.9279) (-9.6351, -11.0184) (-9.8039, -11.0884) knots 0 0 0 1 2 2 2
  spline S183 degree 2 poles (-9.8039, -11.0884) (-9.948, -11.1461) (-10.2156, -11.3107) (-10.2979, -11.3684) knots 0 0 0 1 2 2 2
  line L194 (-10.2979, -11.3684) -> (-10.335, -11.3684)
  line L195 (-10.335, -11.3684) -> (-10.335, -10.6438)
  spline S184 degree 2 poles (-10.335, -10.6438) (-10.125, -10.5409) (-9.3717, -10.3392) (-9.0341, -10.3392) knots 0 0 0 1 2 2 2
  spline S185 degree 2 poles (-9.0341, -10.3392) (-8.3219, -10.3392) (-7.5191, -11.0925) (-7.5191, -11.7347) knots 0 0 0 1 2 2 2
  spline S186 degree 2 poles (-7.5191, -11.7347) (-7.5191, -12.0353) (-7.6591, -12.5375) (-7.7826, -12.7516) knots 0 0 0 1 2 2 2
  spline S187 degree 2 poles (-7.7826, -12.7516) (-7.9061, -12.9739) (-8.2643, -13.4102) (-8.4619, -13.6202) knots 0 0 0 1 2 2 2
  spline S188 degree 2 poles (-8.4619, -13.6202) (-8.783, -13.9701) (-9.5693, -14.7194) (-9.8039, -14.9375) knots 0 0 0 1 2 2 2
  line L196 (-9.8039, -14.9375) -> (-7.3092, -14.9375)
  line L197 (-7.3092, -14.9375) -> (-7.3092, -15.5262)
  line L198 (-3.4395, -11.2078) -> (-5.6378, -15.5262)
  line L199 (-5.6378, -15.5262) -> (-6.3623, -15.5262)
  line L200 (-6.3623, -15.5262) -> (-4.0405, -11.0431)
  line L201 (-4.0405, -11.0431) -> (-6.6629, -11.0431)
  line L202 (-6.6629, -11.0431) -> (-6.6629, -10.4462)
  line L203 (-6.6629, -10.4462) -> (-3.4395, -10.4462)
  line L204 (-3.4395, -10.4462) -> (-3.4395, -11.2078)
  spline S189 degree 2 poles (0.2614, -13.9125) (0.2614, -14.2789) (0.0268, -14.9046) (-0.1873, -15.1351) knots 0 0 0 1 2 2 2
  spline S190 degree 2 poles (-0.1873, -15.1351) (-0.4014, -15.3657) (-1.0395, -15.6333) (-1.4347, -15.6333) knots 0 0 0 1 2 2 2
  spline S191 degree 2 poles (-1.4347, -15.6333) (-1.7969, -15.6333) (-2.505, -15.4727) (-2.7644, -15.3451) knots 0 0 0 1 2 2 2
  line L205 (-2.7644, -15.3451) -> (-2.7644, -14.6247)
  line L206 (-2.7644, -14.6247) -> (-2.715, -14.6247)
  spline S192 degree 2 poles (-2.715, -14.6247) (-2.6367, -14.6823) (-2.3445, -14.8305) (-2.1674, -14.8964) knots 0 0 0 1 2 2 2
  spline S193 degree 2 poles (-2.1674, -14.8964) (-1.9657, -14.9664) (-1.6323, -15.0446) (-1.4223, -15.0446) knots 0 0 0 1 2 2 2
  spline S194 degree 2 poles (-1.4223, -15.0446) (-1.2165, -15.0446) (-0.8295, -14.8964) (-0.6895, -14.7358) knots 0 0 0 1 2 2 2
  spline S195 degree 2 poles (-0.6895, -14.7358) (-0.5619, -14.5835) (-0.4302, -14.1801) (-0.4302, -13.9084) knots 0 0 0 1 2 2 2
  spline S196 degree 2 poles (-0.4302, -13.9084) (-0.4302, -13.6367) (-0.5784, -13.2909) (-0.7184, -13.1756) knots 0 0 0 1 2 2 2
  spline S197 degree 2 poles (-0.7184, -13.1756) (-0.8624, -13.048) (-1.2906, -12.9409) (-1.5499, -12.9409) knots 0 0 0 1 2 2 2
  spline S198 degree 2 poles (-1.5499, -12.9409) (-1.8299, -12.9409) (-2.3856, -13.0274) (-2.5544, -13.0644) knots 0 0 0 1 2 2 2
  line L207 (-2.5544, -13.0644) -> (-2.5544, -10.4462)
  line L208 (-2.5544, -10.4462) -> (0.2326, -10.4462)
  line L209 (0.2326, -10.4462) -> (0.2326, -11.0431)
  line L210 (0.2326, -11.0431) -> (-1.8999, -11.0431)
  line L211 (-1.8999, -11.0431) -> (-1.8999, -12.3975)
  spline S199 degree 2 poles (-1.8999, -12.3975) (-1.7764, -12.3811) (-1.5376, -12.3687) (-1.4388, -12.3687) knots 0 0 0 1 2 2 2
  spline S200 degree 2 poles (-1.4388, -12.3687) (-1.0477, -12.3687) (-0.5084, -12.4963) (-0.2614, -12.6857) knots 0 0 0 1 2 2 2
  spline S201 degree 2 poles (-0.2614, -12.6857) (-0.0103, -12.8751) (0.2614, -13.4514) (0.2614, -13.9125) knots 0 0 0 1 2 2 2
  line L212 (1.7558, -10.2198) -> (1.6076, -12.1958)
  line L213 (1.6076, -12.1958) -> (1.1588, -12.1958)
  line L214 (1.1588, -12.1958) -> (1.0106, -10.2198)
  line L215 (1.0106, -10.2198) -> (1.7558, -10.2198)
  line L216 (3.0402, -10.2198) -> (2.892, -12.1958)
  line L217 (2.892, -12.1958) -> (2.4433, -12.1958)
  line L218 (2.4433, -12.1958) -> (2.2951, -10.2198)
  line L219 (2.2951, -10.2198) -> (3.0402, -10.2198)
  line L220 (9.808, -10.4462) -> (8.0584, -15.5262)
  line L221 (8.0584, -15.5262) -> (7.3298, -15.5262)
  line L222 (7.3298, -15.5262) -> (5.5802, -10.4462)
  line L223 (5.5802, -10.4462) -> (6.3047, -10.4462)
  line L224 (6.3047, -10.4462) -> (7.7126, -14.6658)
  line L225 (7.7126, -14.6658) -> (9.1205, -10.4462)
  line L226 (9.1205, -10.4462) -> (9.808, -10.4462)
  spline S202 degree 2 poles (13.369, -12.9862) (13.369, -14.353) (12.5744, -15.6333) (11.747, -15.6333) knots 0 0 0 1 2 2 2
  spline S203 degree 2 poles (11.747, -15.6333) (10.9072, -15.6333) (10.1209, -14.3283) (10.1209, -12.9903) knots 0 0 0 1 2 2 2
  spline S204 degree 2 poles (10.1209, -12.9903) (10.1209, -11.6154) (10.9154, -10.3433) (11.747, -10.3433) knots 0 0 0 1 2 2 2
  spline S205 degree 2 poles (11.747, -10.3433) (12.5827, -10.3433) (13.369, -11.6606) (13.369, -12.9862) knots 0 0 0 1 2 2 2
  spline S206 degree 2 poles (12.4962, -14.5341) (12.595, -14.283) (12.6774, -13.509) (12.6774, -12.9862) knots 0 0 0 1 2 2 2
  spline S207 degree 2 poles (12.6774, -12.9862) (12.6774, -12.4634) (12.595, -11.6936) (12.4921, -11.4342) knots 0 0 0 1 2 2 2
  spline S208 degree 2 poles (12.4921, -11.4342) (12.3892, -11.1749) (12.031, -10.9073) (11.747, -10.9073) knots 0 0 0 1 2 2 2
  spline S209 degree 2 poles (11.747, -10.9073) (11.4629, -10.9073) (11.0965, -11.1749) (10.9895, -11.4425) knots 0 0 0 1 2 2 2
  spline S210 degree 2 poles (10.9895, -11.4425) (10.8866, -11.7018) (10.8125, -12.4922) (10.8125, -12.9903) knots 0 0 0 1 2 2 2
  spline S211 degree 2 poles (10.8125, -12.9903) (10.8125, -13.5255) (10.8784, -14.2418) (10.9854, -14.5217) knots 0 0 0 1 2 2 2
  spline S212 degree 2 poles (10.9854, -14.5217) (11.0842, -14.7852) (11.4506, -15.0693) (11.747, -15.0693) knots 0 0 0 1 2 2 2
  spline S213 degree 2 poles (11.747, -15.0693) (12.0269, -15.0693) (12.3933, -14.8017) (12.4962, -14.5341) knots 0 0 0 1 2 2 2
  spline S214 degree 2 poles (15.3903, -10.9279) (15.205, -10.9279) (14.8386, -11.0184) (14.6616, -11.0884) knots 0 0 0 1 2 2 2
  spline S215 degree 2 poles (14.6616, -11.0884) (14.4969, -11.1584) (14.2541, -11.3066) (14.1594, -11.3725) knots 0 0 0 1 2 2 2
  line L227 (14.1594, -11.3725) -> (14.1182, -11.3725)
  line L228 (14.1182, -11.3725) -> (14.1182, -10.6521)
  spline S216 degree 2 poles (14.1182, -10.6521) (14.3405, -10.5327) (15.1021, -10.3392) (15.4438, -10.3392) knots 0 0 0 1 2 2 2
  spline S217 degree 2 poles (15.4438, -10.3392) (15.7896, -10.3392) (16.3042, -10.4792) (16.5141, -10.6274) knots 0 0 0 1 2 2 2
  spline S218 degree 2 poles (16.5141, -10.6274) (16.7364, -10.7879) (16.967, -11.2531) (16.967, -11.566) knots 0 0 0 1 2 2 2
  spline S219 degree 2 poles (16.967, -11.566) (16.967, -11.9859) (16.4153, -12.6198) (16.0283, -12.7022) knots 0 0 0 1 2 2 2
  line L229 (16.0283, -12.7022) -> (16.0283, -12.7516)
  spline S220 degree 2 poles (16.0283, -12.7516) (16.1889, -12.7845) (16.5553, -12.9327) (16.7117, -13.0809) knots 0 0 0 1 2 2 2
  spline S221 degree 2 poles (16.7117, -13.0809) (16.8682, -13.225) (17.0658, -13.6861) (17.0658, -14.0195) knots 0 0 0 1 2 2 2
  spline S222 degree 2 poles (17.0658, -14.0195) (17.0658, -14.3612) (16.8311, -14.9417) (16.617, -15.164) knots 0 0 0 1 2 2 2
  spline S223 degree 2 poles (16.617, -15.164) (16.3947, -15.3945) (15.7649, -15.6333) (15.3656, -15.6333) knots 0 0 0 1 2 2 2
  spline S224 degree 2 poles (15.3656, -15.6333) (14.9827, -15.6333) (14.2335, -15.448) (13.9782, -15.3204) knots 0 0 0 1 2 2 2
  line L230 (13.9782, -15.3204) -> (13.9782, -14.6)
  line L231 (13.9782, -14.6) -> (14.0276, -14.6)
  spline S225 degree 2 poles (14.0276, -14.6) (14.2417, -14.7564) (14.9662, -15.0446) (15.3244, -15.0446) knots 0 0 0 1 2 2 2
  spline S226 degree 2 poles (15.3244, -15.0446) (15.5343, -15.0446) (15.9542, -14.9128) (16.0942, -14.7605) knots 0 0 0 1 2 2 2
  spline S227 degree 2 poles (16.0942, -14.7605) (16.2301, -14.6082) (16.3741, -14.2459) (16.3741, -13.9701) knots 0 0 0 1 2 2 2
  spline S228 degree 2 poles (16.3741, -13.9701) (16.3741, -13.6943) (16.2136, -13.3361) (16.0695, -13.2332) knots 0 0 0 1 2 2 2
  spline S229 degree 2 poles (16.0695, -13.2332) (15.9254, -13.1303) (15.5343, -13.0521) (15.3038, -13.0521) knots 0 0 0 1 2 2 2
  line L232 (15.3038, -13.0521) -> (15.0156, -13.0521)
  line L233 (15.0156, -13.0521) -> (15.0156, -12.4881)
  line L234 (15.0156, -12.4881) -> (15.2421, -12.4881)
  spline S230 degree 2 poles (15.2421, -12.4881) (15.699, -12.4881) (16.2753, -12.0517) (16.2753, -11.6359) knots 0 0 0 1 2 2 2
  spline S231 degree 2 poles (16.2753, -11.6359) (16.2753, -11.4425) (16.1271, -11.1666) (16.0078, -11.0843) knots 0 0 0 1 2 2 2
  spline S232 degree 2 poles (16.0078, -11.0843) (15.8801, -10.9979) (15.5673, -10.9279) (15.3903, -10.9279) knots 0 0 0 1 2 2 2
  spline S233 degree 2 poles (23.3684, -11.9776) (23.3684, -12.307) (23.1338, -12.8998) (22.9238, -13.1056) knots 0 0 0 1 2 2 2
  spline S234 degree 2 poles (22.9238, -13.1056) (22.6603, -13.365) (21.9482, -13.6325) (21.4047, -13.6325) knots 0 0 0 1 2 2 2
  line L235 (21.4047, -13.6325) -> (20.8325, -13.6325)
  line L236 (20.8325, -13.6325) -> (20.8325, -15.5262)
  line L237 (20.8325, -15.5262) -> (20.1574, -15.5262)
  line L238 (20.1574, -15.5262) -> (20.1574, -10.4462)
  line L239 (20.1574, -10.4462) -> (21.4336, -10.4462)
  spline S235 degree 2 poles (21.4336, -10.4462) (21.8864, -10.4462) (22.5204, -10.5944) (22.7633, -10.7632) knots 0 0 0 1 2 2 2
  spline S236 degree 2 poles (22.7633, -10.7632) (23.0473, -10.9567) (23.3684, -11.5536) (23.3684, -11.9776) knots 0 0 0 1 2 2 2
  spline S237 degree 2 poles (22.6645, -11.9982) (22.6645, -11.7347) (22.4833, -11.3478) (22.2981, -11.2243) knots 0 0 0 1 2 2 2
  spline S238 degree 2 poles (22.2981, -11.2243) (22.1375, -11.1172) (21.7094, -11.0308) (21.3924, -11.0308) knots 0 0 0 1 2 2 2
  line L240 (21.3924, -11.0308) -> (20.8325, -11.0308)
  line L241 (20.8325, -11.0308) -> (20.8325, -13.0562)
  line L242 (20.8325, -13.0562) -> (21.2936, -13.0562)
  spline S239 degree 2 poles (21.2936, -13.0562) (21.7053, -13.0562) (22.2116, -12.9245) (22.3763, -12.7516) knots 0 0 0 1 2 2 2
  spline S240 degree 2 poles (22.3763, -12.7516) (22.5286, -12.5993) (22.6645, -12.2411) (22.6645, -11.9982) knots 0 0 0 1 2 2 2
  line L243 (27.6951, -10.4462) -> (25.9455, -15.5262)
  line L244 (25.9455, -15.5262) -> (25.2168, -15.5262)
  line L245 (25.2168, -15.5262) -> (23.4672, -10.4462)
  line L246 (23.4672, -10.4462) -> (24.1918, -10.4462)
  line L247 (24.1918, -10.4462) -> (25.5997, -14.6658)
  line L248 (25.5997, -14.6658) -> (27.0076, -10.4462)
  line L249 (27.0076, -10.4462) -> (27.6951, -10.4462)
  spline S241 degree 2 poles (31.256, -12.9862) (31.256, -14.353) (30.4615, -15.6333) (29.634, -15.6333) knots 0 0 0 1 2 2 2
  spline S242 degree 2 poles (29.634, -15.6333) (28.7942, -15.6333) (28.0079, -14.3283) (28.0079, -12.9903) knots 0 0 0 1 2 2 2
  spline S243 degree 2 poles (28.0079, -12.9903) (28.0079, -11.6154) (28.8024, -10.3433) (29.634, -10.3433) knots 0 0 0 1 2 2 2
  spline S244 degree 2 poles (29.634, -10.3433) (30.4697, -10.3433) (31.256, -11.6606) (31.256, -12.9862) knots 0 0 0 1 2 2 2
  spline S245 degree 2 poles (30.3833, -14.5341) (30.4821, -14.283) (30.5644, -13.509) (30.5644, -12.9862) knots 0 0 0 1 2 2 2
  spline S246 degree 2 poles (30.5644, -12.9862) (30.5644, -12.4634) (30.4821, -11.6936) (30.3791, -11.4342) knots 0 0 0 1 2 2 2
  spline S247 degree 2 poles (30.3791, -11.4342) (30.2762, -11.1749) (29.9181, -10.9073) (29.634, -10.9073) knots 0 0 0 1 2 2 2
  spline S248 degree 2 poles (29.634, -10.9073) (29.35, -10.9073) (28.9836, -11.1749) (28.8765, -11.4425) knots 0 0 0 1 2 2 2
  spline S249 degree 2 poles (28.8765, -11.4425) (28.7736, -11.7018) (28.6995, -12.4922) (28.6995, -12.9903) knots 0 0 0 1 2 2 2
  spline S250 degree 2 poles (28.6995, -12.9903) (28.6995, -13.5255) (28.7654, -14.2418) (28.8724, -14.5217) knots 0 0 0 1 2 2 2
  spline S251 degree 2 poles (28.8724, -14.5217) (28.9712, -14.7852) (29.3376, -15.0693) (29.634, -15.0693) knots 0 0 0 1 2 2 2
  spline S252 degree 2 poles (29.634, -15.0693) (29.914, -15.0693) (30.2803, -14.8017) (30.3833, -14.5341) knots 0 0 0 1 2 2 2
  line L250 (34.784, -15.5262) -> (32.3058, -15.5262)
  line L251 (32.3058, -15.5262) -> (32.3058, -15.0075)
  line L252 (32.3058, -15.0075) -> (33.2279, -15.0075)
  line L253 (33.2279, -15.0075) -> (33.2279, -11.603)
  line L254 (33.2279, -11.603) -> (32.3058, -11.603)
  line L255 (32.3058, -11.603) -> (32.3058, -11.1378)
  spline S253 degree 2 poles (32.3058, -11.1378) (32.8286, -11.1378) (33.3226, -10.8414) (33.3555, -10.4298) knots 0 0 0 1 2 2 2
  line L256 (33.3555, -10.4298) -> (33.8824, -10.4298)
  line L257 (33.8824, -10.4298) -> (33.8824, -15.0075)
  line L258 (33.8824, -15.0075) -> (34.784, -15.0075)
  line L259 (34.784, -15.0075) -> (34.784, -15.5262)
  point P0 (0, 25.7175)
  constraints: 2 end point, 2 midpoint, 1 horizontal
emboss "Emboss1" sketch "Sketch4" operation cut depth 2.54 direction (-1, 0, 0) wrap yes faces at (-8.4189, 9.5085, -38.4175)
sketch "Sketch5" plane through (0, 0, 25.7175) normal (0, 0, 1) x (1, 0, 0)
  circle A0 centre (0, 0) radius 4 projected
  constraints: 1 coincident
hole "Hole1" at (0, 0, 25.7175) direction (0, 0, -1) diameter 6.7564 depth 25.4 counterbore diameter 8.509 counterbore depth 12.7 clearance for "Hex Head Bolt" size "1/4" standard "Ansi Unified Screw Threads"
equation "\"d0\" = hexSize"
equation "\"d6\" = printOffset"
equation "\"hexSize\" = 25.4"
equation "\"length\" = 47.625"
equation "\"printOffset\" = 0.09525"
body "Solid1"
